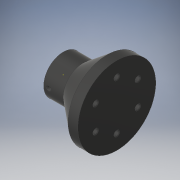
# Autodesk Inventor part: BT405_trajan20_21
Saved by Autodesk Inventor 2022.2 (Build 262287000, 287)
## iProperties
Company: HTBLA Kaindorf
RuleStatus: InUse
Created: 2022-08-22
Part Number: BT405_trajan20_21
Project: Zeichenmaschine_v2
Material: Kunststoff, undurchsichtig Schwarz
Description: zwischenteil_stifte
Document SubType Name: Modeling
Designer: trajan20
Density: 0.952 g/cm^3
Appearance: Glatt - Schwarz
Mass: 139.719 g
Surface Area: 188.748 cm^2
Volume: 146.764 cm^3
AfterDocNew0: iProperties-Editor_aufrufen
Author: jan
Keywords: 2021
Autodesk Inventor part; units mm, degrees
ref_plane "XZ Plane" through (0, 0, 0) normal (0, 1, 0) x (-1, 0, 0)
ref_plane "XY Plane" through (0, 0, 0) normal (0, 0, 1) x (1, 0, 0)
sketch "Skizze3" plane through (0, 0, 0) normal (0, 1, 0) x (-1, 0, 0)
  point P0 (0, 0)
sketch "Skizze4" plane through (0, 0, 0) normal (0, 0, 1) x (1, 0, 0)
  line L0 (0, 0) -> (20, 0)
  line L1 (20, 0) -> (20, 20)
  line L2 (20, 20) -> (40, 45)
  line L3 (40, 45) -> (40, 55)
  line L4 (40, 55) -> (0, 55)
  line L5 (0, 55) -> (0, 0)
  dimension "d5" = 40
  dimension "d6" = 80
  dimension "d7" = 20
  dimension "d8" = 25
  dimension "d9" = 10
  constraints: 12 end point, 3 perpendicular, 1 horizontal, 1 parallel
  measures "d5" diameter of L1 L5
  measures "d6" diameter of L3 L5
  measures "d7" distance of L0.end L1.end
  measures "d8" vertical distance of L2.end L1.end
  measures "d9" distance of L2.end L3.end
revolve "Umdrehung1" add sketch "Skizze4" angle 360 about axis through (0, 55, 0) along (0, -1, 0)
sketch "Skizze5" plane through (0, 55, 0) normal (0, 1, 0) x (1, 0, 0)
  circle A0 centre (0, -25) radius 2.5
  line L0 (0, 56) -> (0, -56) projected
  point P0 (0, 0)
  dimension "d11" = 25
  dimension "d12" = 5
  constraints: 1 centre point, 1 point on line
  measures "d11" distance of point (0, 0) A0.centre
  measures "d12" diameter of A0
extrude "Extrusion3" cut sketch "Skizze5" against normal blind 12
chamfer "Fase1" distance 0.5 angle 45 1 edges at (-2.5, 55, 25)
pattern_circular "Runde Anordnung1" count 6 over 360 about axis through (0, 10, 0) along (0, -1, 0) of "Extrusion3", "Fase1"
ref_plane "Arbeitsebene1" through (20, 0, 0) normal (1, 0, 0) x (0, 1, 0)
sketch "Skizze6" plane through (20, 0, 0) normal (1, 0, 0) x (0, 1, 0)
  line L0 (20, 20) -> (20, -20) projected
  line L1 (0, 20) -> (0, -20) projected
  line L2 (-2.9204, 0) -> (2.9204, 0)
  point P0 (0, 0)
  point P1 (5, 0)
  point P2 (0, 0)
  dimension "d22" = 15
  constraints: 2 end point, 2 midpoint, 1 horizontal, 1 point on line
  measures "d22" distance from line of L0 point (5, 0)
sketch "Skizze7" plane through (0, 0, 0) normal (0, -1, 0) x (1, 0, 0)
  circle A0 centre (0, 0) radius 3
  line L0 (1.199, 2.75) -> (1.199, -2.75)
  point P0 (0, 0)
  dimension "d23" = 6
  dimension "d24" = 5.5
  constraints: 2 end point, 2 point on circle, 1 centre point, 1 coincident, 1 vertical
  measures "d23" diameter of A0
  measures "d24" distance of L0.start L0.end
extrude "Extrusion4" cut sketch "Skizze7" against normal blind 12.2 contours L0 A0 picked at (-0.2225, -0.8366)
hole "Bohrung1" at (20, 5, 0) direction (-1, 0, 0) diameter 4.134 depth 18.801 thread size "M5x0.8" class "6H" standard "ISO Metric profile"
chamfer "Fase2" distance 0.5 angle 45 3 edges at (19.9385, 6.3471, -1.5678) (19.9383, 3.6548, -1.5694) (19.8929, 4.9998, 2.067)
